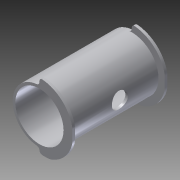
# Autodesk Inventor part: tube-shell
Saved by Autodesk Inventor 2015 (Build 190159000, 159)
## iProperties
Created: 2014-10-04
Part Number: tube-shell
Material: ABS Plastic
Document SubType Name: Modeling
Designer: Adam
Density: 1.06 g/cm^3
Appearance: Smooth - White
Author: Adam
Autodesk Inventor part; units mm, degrees
ref_plane "Work Plane1" through (-11.3089, 3, -83.403141) normal (0, 0, 1) x (1, 0, 0)
sketch "Sketch1" plane through (-11.3089, 3, -83.403141) normal (0, 0, 1) x (1, 0, 0)
  circle A0 centre (11.3089, 0) radius 15.1 construction
  circle A1 centre (11.3089, 0) radius 16.5
  circle A2 centre (11.3089, 0) radius 18.3
  point P0 (11.3089, -3)
  dimension "d0" = 1.8
  dimension "d1" = 33
  constraints: 2 centre point, 2 coincident
  measures "d0" radial gap between concentric circles of A1 A2
  measures "d1" diameter of A1
extrude "Extrusion1" add sketch "Sketch1" along normal blind 85
sketch "Sketch2" plane through (0, 3, -83.403141) normal (0, 0, -1) x (-1, 0, 0)
  circle A0 centre (0, 0) radius 18.3 projected
  circle A1 centre (0, 0) radius 16.5 projected
  point P0 (0, -3)
extrude "Extrusion2" cut sketch "Sketch2" against normal blind 20
ref_plane "Work Plane3" through (18.299967, 3.034617, -83.403141) normal (0.9999982, 0.0018916, 0) x (-0.0018916, 0.9999982, 0)
ref_plane "Work Plane2" through (27.554335, -25.697929, -35.2) normal (0.9999982, 0.0018916, 0) x (0, 0, 1)
sketch "Sketch3" plane through (18.299967, 3.034617, -83.403141) normal (0.9999982, 0.0018916, 0) x (-0.0018916, 0.9999982, 0)
  circle A0 centre (0, 48.203141) radius 10 construction
  ellipse E0 centre (-0.000197, 47.381045) end of major axis (-7.500197, 47.377887) minor radius 1.594171 (-6.479656, 48.181289) -> (6.493506, 48.181289) ccw construction
  circle A1 centre (0, 48.203141) radius 5.5
  point P0 (-2.999995, 83.403141)
  dimension "d6" = 11
  constraints: 1 centre point, 1 coincident, 1 other
  measures "d6" diameter of A1
extrude "Extrusion3" cut sketch "Sketch3" against normal blind 10
sketch "Sketch4" plane through (0, 3, 1.596859) normal (0, 0, 1) x (1, 0, 0)
  arc A0 (22.490937, 4.812249) -> (-0.043507, 22.999959) centre (0, 0) ccw construction
  line L0 (22.508982, -4.727126) -> (22.490937, 4.812249) construction
  arc A1 (19.024484, -12.925517) -> (22.508982, -4.727126) centre (0, 0) ccw construction
  line L1 (19.119065, -62.925428) -> (19.024484, -12.925517) construction
  arc A2 (22.490937, 4.812249) -> (-0.043507, 22.999959) centre (0, 0) ccw
  line L2 (22.490937, 4.812249) -> (22.508982, -4.727126)
  arc A3 (19.024484, -12.925517) -> (22.508982, -4.727126) centre (0, 0) ccw
  line L3 (-0.043507, 22.999959) -> (-0.043507, 18.299948)
  line L4 (19.041582, -21.96402) -> (-5.958374, -22.01131) construction
  arc A4 (6.749808, -21.987271) -> (19.024484, -12.925517) centre (0, 0) ccw
  line L5 (0.041616, -21.999961) -> (6.749808, -21.987271)
  line L6 (0.041616, -21.999961) -> (0.034617, -18.299967)
  line L7 (0.119099, -62.961369) -> (-0.008512, 4.499992) construction
  arc A5 (0.034617, -18.299967) -> (-0.043507, 18.299948) centre (0, 0) ccw
  circle A6 centre (0, 0) radius 16.5 construction
  circle A7 centre (0, 0) radius 18.3 construction
  point P0 (0, -3)
  point P1 (12.954574, -12.925517)
  constraints: 8 end point, 8 point on circle, 4 centre point, 4 coincident, 2 collinear, 2 point on line, 1 concentric, 1 vertical
extrude "Extrusion4" add sketch "Sketch4" against normal blind 1.8
sketch "Sketch5" plane through (0, 3, -63.403141) normal (0, 0, -1) x (-1, 0, 0)
  circle A0 centre (0, 0) radius 16.5 construction
  circle A1 centre (0, 0) radius 18.3 construction
  arc A2 (0.043507, 22.999959) -> (-22.490937, 4.812249) centre (0, 0) ccw
  line L0 (-22.490937, 4.812249) -> (-22.508982, -4.727126)
  arc A3 (-22.508982, -4.727126) -> (-6.749808, -21.987271) centre (0, 0) ccw
  arc A4 (0.043507, 18.299948) -> (-0.034617, -18.299967) centre (0, 0) ccw
  line L1 (0.043507, 18.299948) -> (0.043507, 22.999959)
  line L2 (-6.749808, -21.987271) -> (-0.041616, -21.999961)
  line L3 (-0.041616, -21.999961) -> (-0.034617, -18.299967)
  point P0 (0, -3)
extrude "Extrusion5" add sketch "Sketch5" against normal blind 1.8
ref_plane "Work Plane4" through (0, 3, -62.503141) normal (0, 0, 1) x (1, 0, 0)
fillet "Fillet2" radius 2 4 edges at (0.0346, -15.3, 0.6969) (-0.0435, 21.2999, 0.6969) (0.0346, -15.3, -62.5031) (-0.0435, 21.2999, -62.5031)
fillet "Fillet2" radius 2 4 edges at (0.0416, -19, 0.6969) (-0.0435, 26, 0.6969) (-0.0435, 26, -62.5031) (0.0416, -19, -62.5031)
fillet "Fillet2" radius 10 6 edges at (6.7498, -18.9873, 0.6969) (6.7498, -18.9873, -62.5031) (22.509, -1.7271, 0.6969) (22.4909, 7.8122, 0.6969) (22.509, -1.7271, -62.5031) (22.4909, 7.8122, -62.5031)
ref_plane "Work Plane5" through (-11.3089, 3, 0.696859) normal (0, 0, 1) x (1, 0, 0)
body "Solid1"
